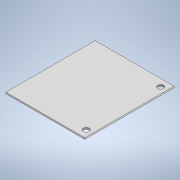
# Autodesk Inventor part: Плата индикации
Saved by Autodesk Inventor 2022 (Build 260153000, 153)
## iProperties
Created: 2022-05-04
Part Number: Плата индикации
Material: Типовые
Document SubType Name: Modeling
Designer: Кочетов.А.И.
Density: 1 g/cm^3
Appearance: По умолчанию
Author: Кочетов.А.И.
Autodesk Inventor part; units mm, degrees
ref_plane "YZ Plane" through (0, 0, 0) normal (1, 0, 0) x (0, 1, 0)
ref_plane "XZ Plane" through (0, 0, 0) normal (0, 1, 0) x (-1, 0, 0)
ref_plane "XY Plane" through (0, 0, 0) normal (0, 0, 1) x (1, 0, 0)
sketch "Эскиз1" plane through (0, 0, 0) normal (0, 1, 0) x (-1, 0, 0)
  line L0 (-26.5, 30) -> (26.5, 30)
  line L1 (26.5, 30) -> (26.5, -30)
  line L2 (26.5, -30) -> (-26.5, -30)
  line L3 (-26.5, -30) -> (-26.5, 30)
  line L4 (-26.5, 30) -> (26.5, -30) construction
  line L5 (26.5, 30) -> (-26.5, -30) construction
  circle A0 centre (-22.5, 25) radius 2
  circle A1 centre (-22.5, -25) radius 2
  line L6 (-26.5, 0) -> (26.5, 0) construction
  point P0 (0, 0)
  dimension "d0" = 60
  dimension "d1" = 53
  dimension "d2" = 4
  dimension "d3" = 50
  dimension "d4" = 4
  constraints: 14 end point, 4 midpoint, 2 centre point, 2 parallel, 1 equal radius, 1 horizontal, 1 perpendicular, 1 symmetric about line
  measures "d0" distance of L0.end L1.end
  measures "d1" distance of L0.start L0.end
  measures "d2" diameter of A0
  measures "d3" distance of A0.centre A1.centre
  measures "d4" distance from line of L3 A0.centre
extrude "Выдавливание1" add sketch "Эскиз1" along normal blind 1
